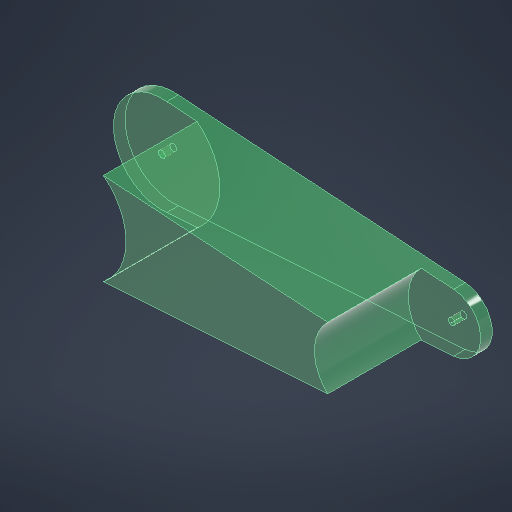
# Autodesk Inventor part: Tibia
Saved by Autodesk Inventor 2026.2 (Build 302298010, 298A)
## iProperties
Created: 2026-07-24
Part Number: Tibia
Material: Generic
Document SubType Name: Modeling
Designer: Entity
Mass: 242.268 g
Surface Area: 330.314 cm^2
Volume: 242.268 cm^3
Density: 1 g/cm^3
Appearance: Clear - Green 1
Author: Entity
Autodesk Inventor part; units mm, degrees
ref_plane "YZ Plane" through (0, 0, 0) normal (1, 0, 0) x (0, 1, 0)
ref_plane "XZ Plane" through (0, 0, 0) normal (0, 1, 0) x (-1, 0, 0)
ref_plane "XY Plane" through (0, 0, 0) normal (0, 0, 1) x (1, 0, 0)
sketch "Sketch1" plane through (0, 0, 0) normal (0, 0, 1) x (1, 0, 0)
  circle A0 centre (0, 0) radius 25
  circle A1 centre (150, 0) radius 15
  line L0 (0, 0) -> (150, 0)
  line L1 (0.7508, 24.9887) -> (150.9983, 14.9667)
  line L2 (0.7508, -24.9887) -> (150.9983, -14.9667)
  point P0 (0.7508, -24.9887)
  point P1 (150.9983, -14.9667)
  point P2 (2.5747, -24.8671)
  point P3 (2.5747, 24.8671)
  dimension "d10" = 15
  dimension "d11" = 25
  dimension "d9" = 150
  constraints: 6 end point, 2 symmetric about line, 1 coincident, 1 horizontal, 7 other
  measures "d9" distance of L0.start L0.end
extrude "Extrusion1" add sketch "Sketch1" along normal blind 6
sketch "Sketch2" plane through (0, 0, 6) normal (0, 0, 1) x (1, 0, 0)
  circle A0 centre (0, 0) radius 1.75
  arc A1 (150.9983, -14.9667) -> (150.9983, 14.9667) centre (150, 0) ccw projected
  circle A2 centre (150, 0) radius 1.75
  point P0 (293.3543, -13.4475)
  point P1 (293.3543, 13.4475)
  point P2 (250.3596, -14.9957)
  point P3 (250.3596, 14.9957)
  dimension "d5" = 3.5
  dimension "d6" = 3.5
  constraints: 2 centre point, 2 coincident, 1 other
  measures "d5" diameter of A0
  measures "d6" diameter of A2
extrude "Extrusion2" cut sketch "Sketch2" against normal blind 6
sketch "Sketch4" plane through (0, 0, 6) normal (0, 0, 1) x (1, 0, 0)
  circle A0 centre (0, 0) radius 12.5
  circle A1 centre (0, 0) radius 1.75 projected
  circle A2 centre (0, 0) radius 30
  circle A3 centre (150, 0) radius 1.75 projected
  circle A4 centre (150, 0) radius 9.913
  arc A5 (150.9983, -14.9667) -> (150.9983, 14.9667) centre (150, 0) ccw projected
  circle A6 centre (150, 0) radius 22.5
  line L0 (150.9983, 14.9667) -> (2.5747, 24.8671) projected
  line L1 (18.2342, 23.8225) -> (134.265, 16.0829)
  line L2 (18.2342, -23.8225) -> (134.265, -16.0829)
  line L3 (2.5747, -24.8671) -> (150.9983, -14.9667) projected
  dimension "d20" = 25
  dimension "d21" = 60
  dimension "d22" = 19.826
  dimension "d23" = 45
  constraints: 4 centre point, 4 coincident, 4 end point, 4 point on circle, 3 point on line
  measures "d20" diameter of A0
  measures "d21" diameter of A2
  measures "d22" diameter of A4
  measures "d23" diameter of A6
extrude "Extrusion4" add sketch "Sketch4" along normal blind 48.5 contours A2 L0 A6 L2
body "Solid1"
